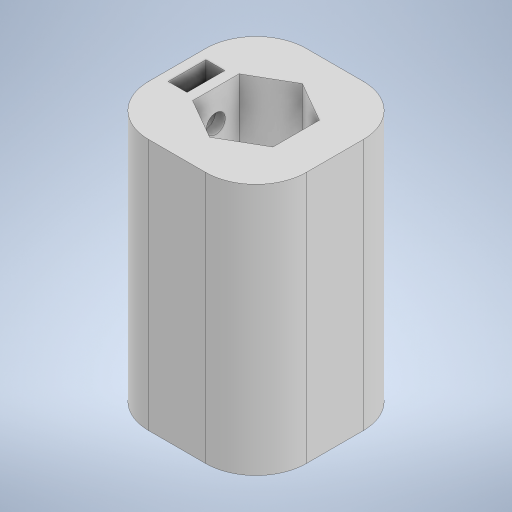
# Autodesk Inventor part: collar
Saved by Autodesk Inventor 2023 (Build 270158000, 158)
## iProperties
Created: 2022-11-01
Part Number: collar
Material: Generic
Document SubType Name: Modeling
Designer: neera
Density: 1 g/cm^3
Appearance: Default
Author: neera
Autodesk Inventor part; units mm, degrees
ref_plane "YZ Plane" through (0, 0, 0) normal (1, 0, 0) x (0, 1, 0)
ref_plane "XZ Plane" through (0, 0, 0) normal (0, 1, 0) x (-1, 0, 0)
ref_plane "XY Plane" through (0, 0, 0) normal (0, 0, 1) x (1, 0, 0)
sketch "Sketch11" plane through (0, 0, 0) normal (0, 1, 0) x (-1, 0, 0)
  arc A0 (2.6519, 1.7) -> (2.6519, -1.7) centre (0, 0) ccw
  line L0 (2.6519, 1.7) -> (2.6519, -1.7)
  line L1 (12.5, 12.5) -> (-12.5, 12.5)
  line L2 (-12.5, 12.5) -> (-12.5, -12.5)
  line L3 (-12.5, -12.5) -> (12.5, -12.5)
  line L4 (12.5, -12.5) -> (12.5, 12.5)
  line L5 (12.5, 12.5) -> (-12.5, -12.5) construction
  line L6 (-12.5, 12.5) -> (12.5, -12.5) construction
  dimension "d45" = 6.3
  dimension "d46" = 3.4
  dimension "d47" = 25
  dimension "d48" = 25
  constraints: 14 end point, 2 midpoint, 2 parallel, 2 point on circle, 1 centre point, 1 coincident, 1 horizontal, 1 perpendicular, 1 vertical
  measures "d45" diameter of A0
  measures "d46" distance of L0.start L0.end
  measures "d47" distance of L3.end L2.end
  measures "d48" distance of L2.end L1.end
extrude "Extrusion8" add sketch "Sketch11" along normal blind 40
sketch "Sketch12" plane through (0, 40, 0) normal (0, 1, 0) x (1, 0, 0)
  line L0 (0, -7.3612) -> (6.375, -3.6806)
  line L1 (6.375, -3.6806) -> (6.375, 3.6806)
  line L2 (6.375, 3.6806) -> (0, 7.3612)
  line L3 (0, 7.3612) -> (-6.375, 3.6806)
  line L4 (-6.375, 3.6806) -> (-6.375, -3.6806)
  line L5 (-6.375, -3.6806) -> (0, -7.3612)
  line L6 (0, -7.3612) -> (0, 0)
  line L7 (0, 0) -> (0, 7.3612)
  point P0 (3.1875, -5.5209)
  dimension "d52" = 120
  dimension "d54" = 12.75
  constraints: 16 end point, 8 equal length, 2 vertical, 1 midpoint
  measures "d52" angle of L2 L3
  measures "d54" distance from line of L3 point (3.187, -5.521)
extrude "Extrusion9" cut sketch "Sketch12" against normal blind 20
sketch "Sketch13" plane through (0, 40, 0) normal (0, 1, 0) x (1, 0, 0)
  line L0 (-7.9375, -3) -> (-10.9375, -3)
  line L1 (-10.9375, -3) -> (-10.9375, 3)
  line L2 (-10.9375, 3) -> (-7.9375, 3)
  line L3 (-7.9375, 3) -> (-7.9375, -3)
  line L4 (-7.9375, -3) -> (-10.9375, 3) construction
  line L5 (-10.9375, -3) -> (-7.9375, 3) construction
  line L6 (-12.5, 12.5) -> (-12.5, -12.5) projected
  point P0 (0, 0)
  point P1 (-9.4375, 0)
  dimension "d57" = 3
  dimension "d58" = 6
  dimension "d59" = 3.0625
  constraints: 12 end point, 2 midpoint, 2 parallel, 1 horizontal, 1 perpendicular
  measures "d57" distance of L1.end L2.end
  measures "d58" distance of L0.end L1.end
  measures "d59" distance from line of L6 point (-9.438, 0)
extrude "Extrusion10" cut sketch "Sketch13" against normal blind 10
sketch "Sketch14" plane through (-7.9375, 40, -3) normal (-1, 0, 0) x (0, 0, 1)
  circle A0 centre (3, -5) radius 1.5
  line L0 (6, 0) -> (6, -10) projected
  line L1 (6, -10) -> (0, -10) projected
  point P0 (3, -40)
  dimension "d62" = 3
  dimension "d63" = 3
  dimension "d64" = 5
  constraints: 1 centre point
  measures "d62" diameter of A0
  measures "d63" distance from line of L0 A0.centre
  measures "d64" distance from line of L1 A0.centre
extrude "Extrusion11" cut sketch "Sketch14" along normal mid plane 10
sketch "Sketch15" plane through (0, 0, 0) normal (0, -1, 0) x (1, 0, 0)
  line L0 (-10.937, -3) -> (-7.937, -3)
  line L1 (-7.937, -3) -> (-7.937, 3)
  line L2 (-7.937, 3) -> (-10.937, 3)
  line L3 (-10.937, 3) -> (-10.937, -3)
  line L4 (-12.5, -12.5) -> (-12.5, 12.5) projected
  point P0 (0, 0)
  point P1 (-9.437, 3)
  dimension "d67" = 3
  dimension "d68" = 6
  dimension "d69" = 4.563
  dimension "d70" = 3
  constraints: 8 end point, 2 parallel, 1 horizontal, 1 midpoint, 1 perpendicular
  measures "d67" distance between parallel lines of L1 L3
  measures "d68" distance from line of L0 point (-9.437, 3)
  measures "d69" distance between parallel lines of L4 L1
  measures "d70" distance from line of point (0, 0) L2
extrude "Extrusion12" cut sketch "Sketch15" against normal blind 10
sketch "Sketch16" plane through (-7.937, 0, -3) normal (-1, 0, 0) x (0, 0, 1)
  circle A0 centre (3, 5) radius 1.5
  line L0 (6, 0) -> (6, 10) projected
  line L1 (-9.5, 0) -> (15.5, 0) projected
  point P0 (3, 0)
  dimension "d73" = 3
  dimension "d74" = 3
  dimension "d75" = 5
  constraints: 1 centre point
  measures "d73" diameter of A0
  measures "d74" distance from line of A0.centre L0
  measures "d75" distance from line of L1 A0.centre
extrude "Extrusion13" cut sketch "Sketch16" along normal blind 10 and the other way blind 6
fillet "Fillet1" radius 8 4 edges at (12.5, 20, -12.5) (12.5, 20, 12.5) (-12.5, 20, -12.5) (-12.5, 20, 12.5)
body "Solid3"
